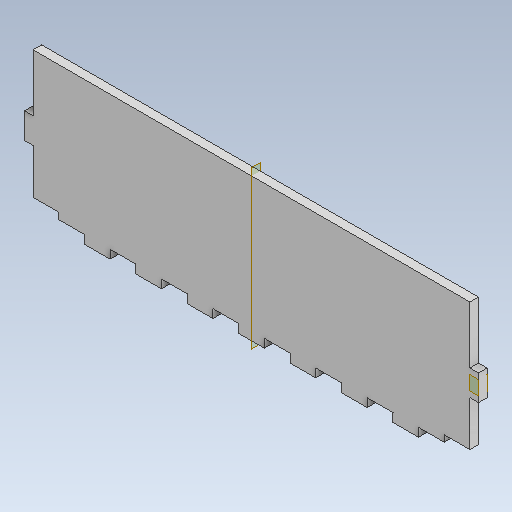
# Autodesk Inventor part: wooden_bottom
Saved by Autodesk Inventor 2020 (Build 240168000, 168)
## iProperties
Created: 2019-07-24
Part Number: wooden_bottom
Material: Generic
Document SubType Name: Modeling
Designer: erwin
Density: 1 g/cm^3
Appearance: Default
Author: erwin
Autodesk Inventor part; units mm, degrees
ref_plane "YZ Plane" through (0, 0, 0) normal (1, 0, 0) x (0, 1, 0)
ref_plane "XZ Plane" through (0, 0, 0) normal (0, 1, 0) x (-1, 0, 0)
ref_plane "XY Plane" through (0, 0, 0) normal (0, 0, 1) x (1, 0, 0)
ref_plane "Work Plane1" through (0, 0, 0) normal (0, 0, 1) x (1, 0, 0)
ref_plane "Work Plane2" through (0, 0, 0) normal (0, 0, 1) x (1, 0, 0)
ref_plane "Work Plane3" through (0, -36, 12) normal (0, 0, -1) x (-1, 0, 0)
ref_plane "Work Plane4" through (0, 0, 0) normal (0, 0, 1) x (1, 0, 0)
sketch "Sketch2" plane through (0, 0, 0) normal (0, 0, 1) x (1, 0, 0)
  line L0 (0, -120) -> (-12, -120)
  line L1 (-12, -120) -> (-12, -36)
  line L2 (-12, -36) -> (0, -36)
  line L3 (0, 0) -> (0, -36)
  line L4 (0, 0) -> (-12, 0)
  line L5 (-12, 0) -> (-12, 102.2276)
  line L6 (-12, 102.2276) -> (0, 102.2276)
  line L7 (0, 102.2276) -> (0, 0)
  line L8 (0, -36) -> (0, -120)
  line L9 (-12, -36) -> (-12, 0)
  line L10 (-12, -112.5877) -> (-42, -112.5877)
  line L11 (-42, -112.5877) -> (-42, -108)
  line L12 (-48, -108) -> (-42, -108)
  line L13 (-84, -108) -> (-48, -108)
  line L14 (-120, -108) -> (-84, -108)
  line L15 (-156, -108) -> (-120, -108)
  line L16 (-192, -108) -> (-156, -108)
  line L17 (-228, -108) -> (-192, -108)
  line L18 (-264, -108) -> (-228, -108)
  line L19 (-300, -108) -> (-264, -108)
  line L20 (-336, -108) -> (-300, -108)
  line L21 (-372, -108) -> (-336, -108)
  line L22 (-408, -108) -> (-372, -108)
  line L23 (-444, -108) -> (-408, -108)
  line L24 (-480, -108) -> (-444, -108)
  line L25 (-516, -108) -> (-480, -108)
  line L26 (-552, -108) -> (-516, -108)
  line L27 (-588, -108) -> (-552, -108)
  line L28 (-624, -108) -> (-588, -108)
  line L29 (-624, -120) -> (-624, -108)
  line L30 (-588, -120) -> (-624, -120)
  line L31 (-588, -120) -> (-588, -108)
  line L32 (-12, -112.5877) -> (-12, -120)
  line L33 (-12, -102.4451) -> (-12, -112.5877)
  line L34 (-42, -102.4451) -> (-12, -102.4451)
  line L35 (-42, -108) -> (-42, -102.4451)
  line L36 (-48, -108) -> (-48, -120)
  line L37 (-12, -120) -> (-48, -120)
  line L38 (-84, -120) -> (-84, -108)
  line L39 (-48, -120) -> (-84, -120)
  line L40 (-120, -108) -> (-120, -120)
  line L41 (-84, -120) -> (-120, -120)
  line L42 (-156, -120) -> (-156, -108)
  line L43 (-120, -120) -> (-156, -120)
  line L44 (-192, -108) -> (-192, -120)
  line L45 (-156, -120) -> (-192, -120)
  line L46 (-228, -120) -> (-228, -108)
  line L47 (-192, -120) -> (-228, -120)
  line L48 (-264, -108) -> (-264, -120)
  line L49 (-228, -120) -> (-264, -120)
  line L50 (-300, -120) -> (-300, -108)
  line L51 (-264, -120) -> (-300, -120)
  line L52 (-336, -108) -> (-336, -120)
  line L53 (-300, -120) -> (-336, -120)
  line L54 (-372, -120) -> (-372, -108)
  line L55 (-336, -120) -> (-372, -120)
  line L56 (-408, -108) -> (-408, -120)
  line L57 (-372, -120) -> (-408, -120)
  line L58 (-444, -120) -> (-444, -108)
  line L59 (-408, -120) -> (-444, -120)
  line L60 (-480, -108) -> (-480, -120)
  line L61 (-444, -120) -> (-480, -120)
  line L62 (-516, -120) -> (-516, -108)
  line L63 (-480, -120) -> (-516, -120)
  line L64 (-552, -108) -> (-552, -120)
  line L65 (-516, -120) -> (-552, -120)
  line L66 (-552, -120) -> (-588, -120)
  line L67 (-624, -108) -> (-12, -108)
  line L68 (-12, -108) -> (-12, 80)
  line L69 (-12, 80) -> (-624, 80)
  line L70 (-624, 80) -> (-624, -108)
  line L71 (-624, 80) -> (-12, 80) projected
  line L72 (-318, 80) -> (-318, -65.4515) construction
  line L73 (-624, -36) -> (-636, -36)
  line L74 (-636, 0) -> (-636, -36)
  line L75 (-636, 0) -> (-624, 0)
  line L76 (-624, -36) -> (-624, 0)
  dimension "d0" = 306
  dimension "d1" = 306
  constraints: 152 end point, 41 horizontal, 28 vertical, 4 symmetric about line, 2 parallel, 2 point on line, 1 midpoint, 1 perpendicular, 46 other
  measures "d0" distance between parallel lines of L70 L72
  measures "d1" distance between parallel lines of L68 L72
extrude "Extrusion1" add sketch "Sketch2" along normal blind 12 contours L2 L9 L4 L3 | L1 L34 L35 L12 L13 L14 L15 L16 L17 L18 L19 L20 L21 L22 L23 L24 L25 L26 L27 L28 L70 L69 L5 L9 | L41 L40 L14 L38 | L45 L44 L16 L42 | L70 L73 L74 L75 | L49 L48 L18 L46 | L53 L52 L20 L50 | L26 L62 L65 L64 | L57 L56 L22 L54 | L24 L58 L61 L60
sketch "Sketch4" plane through (0, 0, 12) normal (0, 0, 1) x (1, 0, 0)
  line L0 (-48, -98.9808) -> (-12, -98.9808) projected
  line L1 (-48, -428.0704) -> (-48, -98.9808) projected
  line L2 (-12, 80) -> (-624, 80) projected
  line L3 (-624, 80) -> (-624, 0) projected
  line L4 (-624, 0) -> (-636, 0) projected
  line L5 (-636, 0) -> (-636, -36) projected
  line L6 (-636, -36) -> (-624, -36) projected
  line L7 (-624, -36) -> (-624, -108) projected
  line L8 (-624, -108) -> (-552, -108) projected
  line L9 (-552, -108) -> (-552, -120) projected
  line L10 (-552, -120) -> (-516, -120) projected
  line L11 (-516, -120) -> (-516, -108) projected
  line L12 (-516, -108) -> (-480, -108) projected
  line L13 (-480, -108) -> (-480, -120) projected
  line L14 (-480, -120) -> (-444, -120) projected
  line L15 (-444, -120) -> (-444, -108) projected
  line L16 (-444, -108) -> (-408, -108) projected
  line L17 (-408, -108) -> (-408, -120) projected
  line L18 (-408, -120) -> (-372, -120) projected
  line L19 (-372, -120) -> (-372, -108) projected
  line L20 (-372, -108) -> (-336, -108) projected
  line L21 (-336, -108) -> (-336, -120) projected
  line L22 (-336, -120) -> (-300, -120) projected
  line L23 (-300, -120) -> (-300, -108) projected
  line L24 (-300, -108) -> (-264, -108) projected
  line L25 (-264, -108) -> (-264, -120) projected
  line L26 (-264, -120) -> (-228, -120) projected
  line L27 (-228, -120) -> (-228, -108) projected
  line L28 (-228, -108) -> (-192, -108) projected
  line L29 (-192, -108) -> (-192, -120) projected
  line L30 (-192, -120) -> (-156, -120) projected
  line L31 (-156, -120) -> (-156, -108) projected
  line L32 (-156, -108) -> (-120, -108) projected
  line L33 (-120, -108) -> (-120, -120) projected
  line L34 (-120, -120) -> (-84, -120) projected
  line L35 (-84, -120) -> (-84, -108) projected
  line L36 (-84, -108) -> (-42, -108) projected
  line L37 (-42, -108) -> (-42, -102.4451) projected
  line L38 (-42, -102.4451) -> (-12, -102.4451) projected
  line L39 (-12, -102.4451) -> (-12, -36) projected
  line L40 (-12, -36) -> (0, -36) projected
  line L41 (0, -36) -> (0, 0) projected
  line L42 (0, 0) -> (-12, 0) projected
  line L43 (-12, 0) -> (-12, 80) projected
  point P0 (-48, -108)
extrude "Extrusion2" cut sketch "Sketch4" against normal blind 12 contours L0 L39 L38 L37 L36 L1
ref_plane "Work Plane5" through (-318, -36, 0) normal (-1, 0, 0) x (0, 0, 1)
mirror "Mirror1" about plane through (-318, -36, 0) normal (-1, 0, 0) of "Extrusion2"
delete faces "Delete Face1" heal no whole lump yes faces at (-594, -106.1484, 8)
equation "\"d0\" = d1"
body "Solid1"
